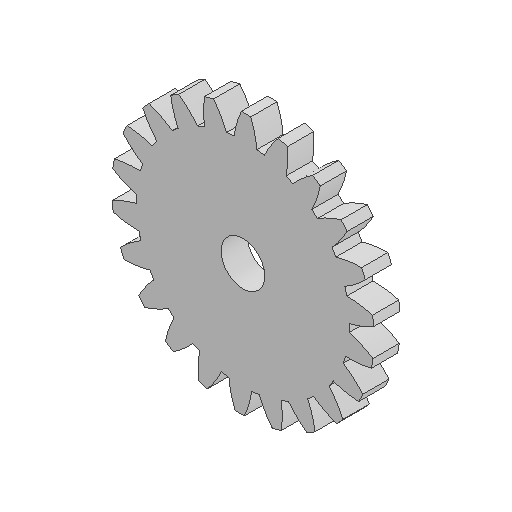
# Autodesk Inventor part: team29
Saved by Autodesk Inventor 2023 (Build 270158000, 158)
## iProperties
Created: 2023-02-27
Part Number: team29
Material: Generic
Document SubType Name: Modeling
Designer: Ethan Ko
Density: 1 g/cm^3
Appearance: Default
Author: Ethan Ko
Autodesk Inventor part; units mm, degrees
ref_plane "YZ Plane" through (0, 0, 0) normal (1, 0, 0) x (0, 1, 0)
ref_plane "XZ Plane" through (0, 0, 0) normal (0, 1, 0) x (-1, 0, 0)
ref_plane "XY Plane" through (0, 0, 0) normal (0, 0, 1) x (1, 0, 0)
sketch "Sketch2" plane through (0, 0, 0) normal (0, 0, 1) x (1, 0, 0)
  arc A0 (-0.6545, -2.0948) -> (-1.4368, -1.7142) centre (-6.3746, -12.8566) ccw
  arc A1 (-1.4368, -1.7142) -> (-1.2915, 1.2546) centre (-12.1132, 0.2962) ccw
  arc A2 (-1.2915, 1.2546) -> (-2.3112, 1.5813) centre (-6.3746, -12.8566) ccw
  arc A3 (-2.3112, 1.5813) -> (-3.9181, -0.9192) centre (5.9388, -5.4873) ccw
  arc A4 (-3.9181, -0.9192) -> (-4.776, -0.7744) centre (-6.3746, -12.8566) ccw
  arc A5 (-4.776, -0.7744) -> (-5.473, 2.1151) centre (-15.5863, -1.8534) ccw
  arc A6 (-5.473, 2.1151) -> (-6.5434, 2.1412) centre (-6.3746, -12.8566) ccw
  arc A7 (-6.5434, 2.1412) -> (-7.3808, -0.7107) centre (3.3639, -2.3167) ccw
  arc A8 (-7.3808, -0.7107) -> (-8.2447, -0.8134) centre (-6.3746, -12.8566) ccw
  arc A9 (-8.2447, -0.8134) -> (-9.7275, 1.7626) centre (-18.3131, -4.8943) ccw
  arc A10 (-9.7275, 1.7626) -> (-10.7619, 1.4862) centre (-6.3746, -12.8566) ccw
  arc A11 (-10.7619, 1.4862) -> (-10.7619, -1.4862) centre (0, 0) ccw
  arc A12 (-10.7619, -1.4862) -> (-11.5619, -1.8281) centre (-6.3746, -12.8566) ccw
  arc A13 (-11.5619, -1.8281) -> (-13.7104, 0.2258) centre (-20.0728, -8.5804) ccw
  arc A14 (-13.7104, 0.2258) -> (-14.625, -0.3309) centre (-6.3746, -12.8566) ccw
  arc A15 (-14.625, -0.3309) -> (-13.7876, -3.1828) centre (-3.8803, 1.2751) ccw
  arc A16 (-13.7876, -3.1828) -> (-14.4588, -3.7363) centre (-6.3746, -12.8566) ccw
  arc A17 (-14.4588, -3.7363) -> (-17.099, -2.3709) centre (-20.7226, -12.6128) ccw
  arc A18 (-17.099, -2.3709) -> (-17.8197, -3.1627) centre (-6.3746, -12.8566) ccw
  arc A19 (-17.8197, -3.1627) -> (-16.2128, -5.6632) centre (-7.9627, 1.4054) ccw
  arc A20 (-16.2128, -5.6632) -> (-16.7009, -6.3833) centre (-6.3746, -12.8566) ccw
  arc A21 (-16.7009, -6.3833) -> (-19.6187, -5.8171) centre (-20.2101, -16.665) ccw
  arc A22 (-19.6187, -5.8171) -> (-20.0872, -6.7798) centre (-6.3746, -12.8566) ccw
  arc A23 (-20.0872, -6.7798) -> (-17.8409, -8.7263) centre (-11.9165, 0.3803) ccw
  arc A24 (-17.8409, -8.7263) -> (-18.1063, -9.5548) centre (-6.3746, -12.8566) ccw
  arc A25 (-18.1063, -9.5548) -> (-21.0655, -9.8335) centre (-18.5767, -20.4087) ccw
  arc A26 (-21.0655, -9.8335) -> (-21.2437, -10.8893) centre (-6.3746, -12.8566) ccw
  arc A27 (-21.2437, -10.8893) -> (-18.54, -12.124) centre (-15.4212, -1.7172) ccw
  arc A28 (-18.54, -12.124) -> (-18.5613, -12.9937) centre (-6.3746, -12.8566) ccw
  arc A29 (-18.5613, -12.9937) -> (-21.3221, -14.0949) centre (-15.9548, -23.5405) ccw
  arc A30 (-21.3221, -14.0949) -> (-21.1957, -15.1581) centre (-6.3746, -12.8566) ccw
  arc A31 (-21.1957, -15.1581) -> (-18.2536, -15.5811) centre (-18.1931, -4.7172) ccw
  arc A32 (-18.2536, -15.5811) -> (-18.029, -16.4216) centre (-6.3746, -12.8566) ccw
  arc A33 (-18.029, -16.4216) -> (-20.3678, -18.2559) centre (-12.5567, -25.8068) ccw
  arc A34 (-19.9469, -19.2405) -> (-17.0049, -18.8174) centre (-20.0075, -8.3766) ccw
  arc A35 (-20.3678, -18.2559) -> (-19.9469, -19.2405) centre (-6.3746, -12.8566) ccw
  arc A36 (-17.0049, -18.8174) -> (-16.5525, -19.5606) centre (-6.3746, -12.8566) ccw
  arc A37 (-16.5525, -19.5606) -> (-18.2798, -21.9796) centre (-8.6578, -27.0239) ccw
  arc A38 (-18.2798, -21.9796) -> (-17.5986, -22.8056) centre (-6.3746, -12.8566) ccw
  arc A39 (-17.5986, -22.8056) -> (-14.8949, -21.5709) centre (-20.7174, -12.3989) ccw
  arc A40 (-14.8949, -21.5709) -> (-14.2515, -22.1565) centre (-6.3746, -12.8566) ccw
  arc A41 (-14.2515, -22.1565) -> (-15.2273, -24.9641) centre (-4.5739, -27.0933) ccw
  arc A42 (-15.2273, -24.9641) -> (-14.341, -25.5648) centre (-6.3746, -12.8566) ccw
  arc A43 (-14.341, -25.5648) -> (-12.0946, -23.6184) centre (-20.2654, -16.4583) ccw
  arc A44 (-12.0946, -23.6184) -> (-11.3123, -23.999) centre (-6.3746, -12.8566) ccw
  arc A45 (-11.3123, -23.999) -> (-11.4576, -26.9678) centre (-0.6359, -26.0093) ccw
  arc A46 (-11.4576, -26.9678) -> (-10.438, -27.2944) centre (-6.3746, -12.8566) ccw
  arc A47 (-10.438, -27.2944) -> (-8.831, -24.794) centre (-18.688, -20.2259) ccw
  arc A48 (-8.831, -24.794) -> (-7.9731, -24.9388) centre (-6.3746, -12.8566) ccw
  arc A49 (-7.9731, -24.9388) -> (-7.2761, -27.8282) centre (2.8372, -23.8598) ccw
  arc A50 (-7.2761, -27.8282) -> (-6.2057, -27.8544) centre (-6.3746, -12.8566) ccw
  arc A51 (-6.2057, -27.8544) -> (-5.3683, -25.0025) centre (-16.113, -23.3964) ccw
  arc A52 (-5.3683, -25.0025) -> (-4.5044, -24.8997) centre (-6.3746, -12.8566) ccw
  arc A53 (-4.5044, -24.8997) -> (-3.0216, -27.4758) centre (5.564, -20.8188) ccw
  arc A54 (-3.0216, -27.4758) -> (-1.9872, -27.1993) centre (-6.3746, -12.8566) ccw
  arc A55 (-1.9872, -27.1993) -> (-1.9872, -24.227) centre (-12.7491, -25.7131) ccw
  arc A56 (-1.9872, -24.227) -> (-1.1872, -23.885) centre (-6.3746, -12.8566) ccw
  arc A57 (-1.1872, -23.885) -> (0.9613, -25.9389) centre (7.3236, -17.1328) ccw
  arc A58 (0.9613, -25.9389) -> (1.8759, -25.3823) centre (-6.3746, -12.8566) ccw
  arc A59 (1.8759, -25.3823) -> (1.0385, -22.5303) centre (-8.8688, -26.9883) ccw
  arc A60 (1.0385, -22.5303) -> (1.7097, -21.9769) centre (-6.3746, -12.8566) ccw
  arc A61 (1.7097, -21.9769) -> (4.3499, -23.3423) centre (7.9735, -13.1003) ccw
  arc A62 (4.3499, -23.3423) -> (5.0706, -22.5505) centre (-6.3746, -12.8566) ccw
  arc A63 (5.0706, -22.5505) -> (3.4636, -20.05) centre (-4.7864, -27.1186) ccw
  arc A64 (3.4636, -20.05) -> (3.9517, -19.3298) centre (-6.3746, -12.8566) ccw
  arc A65 (3.9517, -19.3298) -> (6.8696, -19.8961) centre (7.461, -9.0482) ccw
  arc A66 (6.8696, -19.8961) -> (7.3381, -18.9333) centre (-6.3746, -12.8566) ccw
  arc A67 (7.3381, -18.9333) -> (5.0917, -16.9869) centre (-0.8327, -26.0934) ccw
  arc A68 (5.0917, -16.9869) -> (5.3572, -16.1584) centre (-6.3746, -12.8566) ccw
  arc A69 (5.3572, -16.1584) -> (8.3164, -15.8796) centre (5.8276, -5.3045) ccw
  arc A70 (8.3164, -15.8796) -> (8.4946, -14.8239) centre (-6.3746, -12.8566) ccw
  arc A71 (8.4946, -14.8239) -> (5.7909, -13.5891) centre (2.6721, -23.9959) ccw
  arc A72 (5.7909, -13.5891) -> (5.8122, -12.7194) centre (-6.3746, -12.8566) ccw
  arc A73 (5.8122, -12.7194) -> (8.573, -11.6183) centre (3.2057, -2.1727) ccw
  arc A74 (8.573, -11.6183) -> (8.4466, -10.5551) centre (-6.3746, -12.8566) ccw
  arc A75 (8.4466, -10.5551) -> (5.5045, -10.1321) centre (5.444, -20.9959) ccw
  arc A76 (5.5045, -10.1321) -> (5.2799, -9.2916) centre (-6.3746, -12.8566) ccw
  arc A77 (5.2799, -9.2916) -> (7.6186, -7.4572) centre (-0.1924, 0.0936) ccw
  arc A78 (7.6186, -7.4572) -> (7.1978, -6.4727) centre (-6.3746, -12.8566) ccw
  arc A79 (7.1978, -6.4727) -> (4.2557, -6.8957) centre (7.2583, -17.3366) ccw
  arc A80 (4.2557, -6.8957) -> (3.8034, -6.1525) centre (-6.3746, -12.8566) ccw
  arc A81 (3.8034, -6.1525) -> (5.5306, -3.7336) centre (-4.0913, 1.3108) ccw
  arc A82 (5.5306, -3.7336) -> (4.8495, -2.9075) centre (-6.3746, -12.8566) ccw
  arc A83 (4.8495, -2.9075) -> (2.1458, -4.1423) centre (7.9683, -13.3143) ccw
  arc A84 (2.1458, -4.1423) -> (1.5024, -3.5566) centre (-6.3746, -12.8566) ccw
  arc A85 (1.5024, -3.5566) -> (2.4781, -0.749) centre (-8.1752, 1.3801) ccw
  arc A86 (1.5918, -0.1483) -> (-0.6545, -2.0948) centre (7.5162, -9.2549) ccw
  arc A87 (2.4781, -0.749) -> (1.5918, -0.1483) centre (-6.3746, -12.8566) ccw
  circle A88 centre (-6.3746, -12.8566) radius 2.5
  dimension "d9" = 5
  constraints: 176 point on circle, 89 centre point, 1 coincident
  measures "d9" diameter of A88
extrude "Extrusion1" add sketch "Sketch2" along normal blind 3
body "Solid1"
